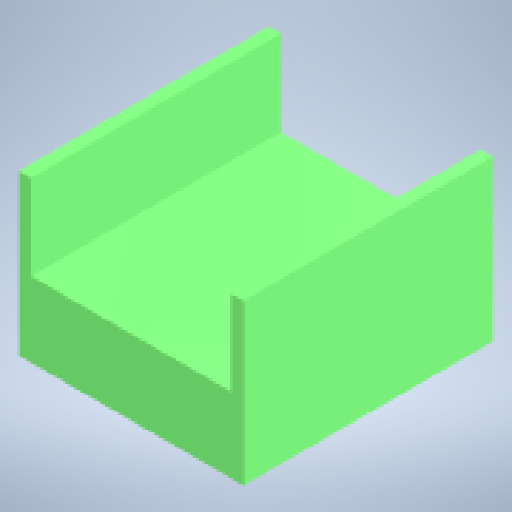
# Autodesk Inventor part: cuscinetto
Saved by Autodesk Inventor 2024 (Build 280153000, 153)
## iProperties
Created: 2023-12-23
Part Number: cuscinetto
Material: Generico
Document SubType Name: Modeling
Designer: Giorgio
Density: 1 g/cm^3
Appearance: Default
Mass: 17.25 g
Surface Area: 70.9 cm^2
Volume: 17.25 cm^3
Author: Giorgio
Autodesk Inventor part; units mm, degrees
ref_plane "YZ Plane" through (0, 0, 0) normal (1, 0, 0) x (0, 1, 0)
ref_plane "XZ Plane" through (0, 0, 0) normal (0, 1, 0) x (-1, 0, 0)
ref_plane "XY Plane" through (0, 0, 0) normal (0, 0, 1) x (1, 0, 0)
sketch "Schizzo1" plane through (0, 0, 0) normal (0, 0, 1) x (1, 0, 0)
  line L0 (-15, 8.4591) -> (-15, -23.5409)
  line L1 (-15, -23.5409) -> (30, -23.5409)
  line L2 (30, -23.5409) -> (30, 8.4591)
  line L3 (30, 8.4591) -> (27.5, 8.4591)
  line L4 (27.5, 8.4591) -> (27.5, -8.5409)
  line L5 (27.5, -8.5409) -> (-12.5, -8.5409)
  line L6 (-12.5, -8.5409) -> (-12.5, 8.4591)
  line L7 (-12.5, 8.4591) -> (-15, 8.4591)
  point P0 (0, 0)
  dimension "d0" = 45
  dimension "d1" = 40
  dimension "d2" = 32
  dimension "d3" = 17
  dimension "d4" = 2.5
  constraints: 16 end point, 6 perpendicular, 1 horizontal, 1 point on line, 1 vertical
  measures "d0" distance of L0.end L1.end
  measures "d1" distance of L4.end L5.end
  measures "d2" distance of L0.start L0.end
  measures "d3" distance of L5.end L6.end
  measures "d4" distance between parallel lines of L0 L6
extrude "Estrusione1" add sketch "Schizzo1" along normal blind 50
equation "\"d4\" = -0.5 * d1 + 0.5 * d0"
